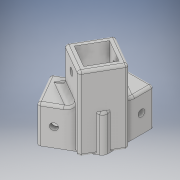
# Autodesk Inventor part: 60_deg_2020_joint
Saved by Autodesk Inventor 2019.4 (Build 234330000, 330)
## iProperties
Created: 2020-01-31
Part Number: 60_deg_2020_joint
Material: Generic
Document SubType Name: Modeling
Designer: Jorian Bruslind
Density: 1 g/cm^3
Appearance: Default
Author: Jorian Bruslind
Autodesk Inventor part; units mm, degrees
ref_plane "YZ Plane" through (0, 0, 0) normal (1, 0, 0) x (0, 1, 0)
ref_plane "XZ Plane" through (0, 0, 0) normal (0, 1, 0) x (-1, 0, 0)
ref_plane "XY Plane" through (0, 0, 0) normal (0, 0, 1) x (1, 0, 0)
sketch "Sketch1" plane through (0, 0, 0) normal (0, 1, 0) x (-1, 0, 0)
  line L0 (0, 0) -> (30, 0)
  line L1 (30, 0) -> (30, -40)
  line L2 (30, -40) -> (0, -40)
  line L3 (0, -40) -> (0, 0)
  line L4 (0, 0) -> (15, -25.9808)
  line L5 (0, 0) -> (30, 0) construction
  line L6 (0, 0) -> (15, -25.9808)
  line L7 (15, -25.9808) -> (49.641, -5.9808)
  line L8 (49.641, -5.9808) -> (34.641, 20)
  line L9 (34.641, 20) -> (0, 0)
  dimension "d1" = 30
  dimension "d2" = 40
  dimension "d3" = 30
  dimension "d4" = 60
  dimension "d5" = 40
  constraints: 20 end point, 6 equal length, 2 horizontal, 2 perpendicular
  measures "d1" distance of L1.end L2.end
  measures "d2" distance of L0.end L1.end
  measures "d3" distance of L0.start L4.end
  measures "d4" angle of L4 L5
  measures "d5" distance of L7.end L4.end
extrude "Extrusion1" add sketch "Sketch1" along normal blind 30
sketch "Sketch9" plane through (-34.641, 0, 20) normal (-0.8660254, 0, 0.5) x (0.5, 0, 0.8660254)
  line L0 (0, 0) -> (0, 15)
  line L1 (0, 0) -> (0, 30) projected
  line L2 (0, 15) -> (-15, 15)
  line L3 (-25.5, 4.5) -> (-4.5, 4.5)
  line L4 (-4.5, 4.5) -> (-4.5, 25.5)
  line L5 (-4.5, 25.5) -> (-25.5, 25.5)
  line L6 (-25.5, 25.5) -> (-25.5, 4.5)
  line L7 (-25.5, 4.5) -> (-4.5, 25.5) construction
  line L8 (-4.5, 4.5) -> (-25.5, 25.5) construction
  dimension "d41" = 15
  dimension "d42" = 21
  dimension "d43" = 21
  constraints: 16 end point, 3 midpoint, 2 parallel, 2 perpendicular
  measures "d41" distance of L0.end L2.end
  measures "d42" distance of L3.start L3.end
  measures "d43" distance of L4.end L3.end
extrude "Extrusion9" cut sketch "Sketch9" against normal blind 25
sketch "Sketch10" plane through (0, 0, -40) normal (0, 0, -1) x (-1, 0, 0)
  line L0 (0, 0) -> (0, 15)
  line L1 (0, 0) -> (0, 30) projected
  line L2 (0, 15) -> (15, 15)
  line L3 (25.5, 4.5) -> (4.5, 4.5)
  line L4 (4.5, 4.5) -> (4.5, 25.5)
  line L5 (4.5, 25.5) -> (25.5, 25.5)
  line L6 (25.5, 25.5) -> (25.5, 4.5)
  line L7 (25.5, 4.5) -> (4.5, 25.5) construction
  line L8 (4.5, 4.5) -> (25.5, 25.5) construction
  dimension "d46" = 15
  dimension "d47" = 21
  dimension "d48" = 21
  constraints: 16 end point, 3 midpoint, 2 parallel, 2 perpendicular
  measures "d46" distance of L0.end L2.end
  measures "d47" distance of L3.start L3.end
  measures "d48" distance of L3.end L4.end
extrude "Extrusion10" cut sketch "Sketch10" against normal blind 25
sketch "Sketch11" plane through (0, 30, 0) normal (0, 1, 0) x (1, 0, 0)
  line L0 (-30, 17.3205) -> (-49.641, 5.9808) projected
  line L1 (0, 0) -> (-30, 17.3205)
  line L2 (-20.4904, 29.1506) -> (5.4904, 14.1506)
  line L3 (5.4904, 14.1506) -> (-9.5096, -11.8301)
  line L4 (-9.5096, -11.8301) -> (-35.4904, 3.1699)
  line L5 (-35.4904, 3.1699) -> (-20.4904, 29.1506)
  line L6 (-20.4904, 29.1506) -> (-9.5096, -11.8301) construction
  line L7 (5.4904, 14.1506) -> (-35.4904, 3.1699) construction
  point P0 (-15, 8.6603)
  dimension "d51" = 30
  dimension "d52" = 30
  constraints: 14 end point, 3 midpoint, 2 parallel, 1 perpendicular
  measures "d51" distance of L2.start L2.end
  measures "d52" distance of L2.end L3.end
extrude "Extrusion11" add sketch "Sketch11" along normal mid plane 60
sketch "Sketch12" plane through (0, 60, 0) normal (0, 1, 0) x (1, 0, 0)
  line L0 (0, 0) -> (0, 4.641) projected
  line L1 (-30, 40) -> (-30, 17.3205) projected
  line L2 (0, 0) -> (-30, 17.3205)
  line L3 (-11.1567, -5.683) -> (-29.3433, 4.817)
  line L4 (-29.3433, 4.817) -> (-18.8433, 23.0035)
  line L5 (-18.8433, 23.0035) -> (-0.6567, 12.5035)
  line L6 (-0.6567, 12.5035) -> (-11.1567, -5.683)
  line L7 (-11.1567, -5.683) -> (-18.8433, 23.0035) construction
  line L8 (-29.3433, 4.817) -> (-0.6567, 12.5035) construction
  point P0 (-15, 8.6603)
  dimension "d55" = 21
  dimension "d56" = 21
  constraints: 14 end point, 3 midpoint, 2 parallel, 1 perpendicular
  measures "d55" distance of L3.start L3.end
  measures "d56" distance of L3.end L4.end
extrude "Extrusion12" cut sketch "Sketch12" against normal blind 25
sketch "Sketch13" plane through (0, 0, 0) normal (1, 0, 0) x (0, 0, -1)
  line L0 (40, 0) -> (40, 30) projected
  line L1 (40, 15) -> (30, 15)
  circle A0 centre (30, 15) radius 2.75
  point P0 (0, 0)
  dimension "d59" = 10
  dimension "d60" = 5.5
  constraints: 2 end point, 1 centre point, 1 coincident, 1 horizontal, 1 midpoint
  measures "d59" distance of L1.start L1.end
  measures "d60" diameter of A0
extrude "Extrusion13" cut sketch "Sketch13" against normal blind 30
sketch "Sketch14" plane through (0, 0, 0) normal (0.5, 0, 0.8660254) x (0.8660254, 0, -0.5)
  line L0 (-40, 4.5) -> (-40, 25.5) projected
  line L1 (-40, 15) -> (-30, 15)
  circle A0 centre (-30, 15) radius 2.75
  point P0 (0, 0)
  dimension "d63" = 10
  dimension "d64" = 5.5
  constraints: 2 end point, 1 centre point, 1 coincident, 1 horizontal, 1 midpoint
  measures "d63" distance of L1.start L1.end
  measures "d64" diameter of A0
extrude "Extrusion14" cut sketch "Sketch14" against normal blind 30
sketch "Sketch15" plane through (-20.4904, 30, -29.1506) normal (0.5, 0, -0.8660254) x (-0.8660254, 0, -0.5)
  line L0 (0, 30) -> (-30, 30) projected
  line L1 (-15, 30) -> (-15, 20)
  circle A0 centre (-15, 20) radius 2.75
  point P0 (-32.3205, -30)
  dimension "d67" = 10
  dimension "d68" = 5.5
  constraints: 2 end point, 1 centre point, 1 coincident, 1 midpoint, 1 vertical
  measures "d67" distance of L1.start L1.end
  measures "d68" diameter of A0
extrude "Extrusion15" cut sketch "Sketch15" against normal blind 30
fillet "Fillet7" radius 5 1 edges at (0, 15, 0)
fillet "Fillet8" radius 5 3 edges at (-10.2452, 30, -23.2356) (-25.2452, 30, 2.7452) (-27.9904, 30, -16.1603)
fillet "Fillet9" radius 5 1 edges at (-30, 15.3893, -17.3205)
fillet "Fillet10" radius 2 10 edges at (-42.141, 30, 7.0096) (-34.641, 15, 20) (-49.641, 15, -5.9808) (-16.4645, 31.4645, 9.5058) (-27.3205, 30, 15.7735) (-33.5621, 30.039, -15.2639) (-30.6699, 30.3775, -17.7073) (-30, 30.039, -21.4337) (-30, 30, -31.3397) (-42.141, 30, -10.3109)
fillet "Fillet11" radius 2 6 edges at (-29.4142, 29.4142, -40) (-30, 14, -40) (-14, 30, -40) (0, 31.4645, -19.0115) (0, 30, -31.547) (0, 15, -40)
fillet "Fillet12" radius 2 2 edges at (-6.7644, 0, 7.0753) (2.7452, 0, -9.3958)
fillet "Fillet13" radius 2 3 edges at (-3.2596, 30, 1.8819) (0, 30, -3.7639) (-0.6699, 30, -0.3868)
fillet "Fillet14" radius 2 4 edges at (-2.0096, 60, -1.1603) (-7.5, 60, -21.6506) (-27.9904, 60, -16.1603) (-22.5, 60, 4.3301)
fillet "Fillet15" radius 2 6 edges at (-34.6902, 59.4142, -3.3843) (-37.4909, 31.4645, -2.6338) (-35.4904, 46.5, -3.1699) (-20.276, 59.4142, -28.3504) (-21.0264, 31.4645, -31.1511) (-20.4904, 46.5, -29.1506)
fillet "Fillet16" radius 2 4 edges at (-9.724, 59.4142, 11.0299) (-9.5096, 30, 11.8301) (4.6902, 59.4142, -13.9362) (5.4904, 30, -14.1506)
body "Solid1"
